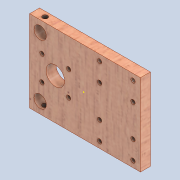
# Autodesk Inventor part: 0005-10-011
Saved by Autodesk Inventor 2020 (Build 240168000, 168)
## iProperties
Created: 2020-12-18
Part Number: 0005-10-011
Material: Wood (Maple)
Document SubType Name: Modeling
Designer: Iulian Bors
Density: 0.67 g/cm^3
Appearance: White Oak - Natural Medium Gloss
Mass: 29.1797 g
Surface Area: 153.939 cm^2
Volume: 43.5518 cm^3
Author: Iulian Bors
Subject: 011
Autodesk Inventor part; units mm, degrees
ref_plane "YZ Plane" through (0, 0, 0) normal (1, 0, 0) x (0, 1, 0)
ref_plane "XZ Plane" through (0, 0, 0) normal (0, 1, 0) x (-1, 0, 0)
ref_plane "XY Plane" through (0, 0, 0) normal (0, 0, 1) x (1, 0, 0)
sketch "Sketch1" plane through (0, 0, 0) normal (0, 0, 1) x (1, 0, 0)
  line L0 (-43.75, 33) -> (43.75, 33)
  line L1 (43.75, 33) -> (43.75, -33)
  line L2 (43.75, -33) -> (-43.75, -33)
  line L3 (-43.75, -33) -> (-43.75, 33)
  point P0 (0, 0)
  point P1 (0, 33)
  point P2 (-43.75, 0)
  dimension "d0" = 87.5
  dimension "d1" = 66
  constraints: 8 end point, 2 midpoint, 2 parallel, 1 horizontal, 1 horizontal alignment, 1 perpendicular, 1 vertical alignment
  measures "d0" distance of L0.start L0.end
  measures "d1" distance of L2.end L0.start
extrude "Extrusion1" add sketch "Sketch1" along normal blind 8
sketch "Sketch4" plane through (0, 0, 8) normal (0, 0, 1) x (1, 0, 0)
  line L0 (43.75, 33) -> (-43.75, 33) projected
  line L1 (-43.75, 33) -> (-43.75, -33) projected
  circle A0 centre (-35.25, 24) radius 5
  circle A1 centre (-35.25, -24) radius 5
  line L2 (-43.75, -33) -> (43.75, -33) projected
  point P0 (0, 0)
  dimension "d27" = 8.5
  dimension "d28" = 9
  dimension "d29" = 10
  dimension "d30" = 9
  constraints: 2 centre point, 1 equal radius, 1 vertical alignment
  measures "d27" distance from line of A0.centre L1
  measures "d28" distance from line of L0 A0.centre
  measures "d29" diameter of A0
  measures "d30" distance from line of L2 A1.centre
extrude "Extrusion4" cut sketch "Sketch4" against normal through all
sketch "Sketch5" plane through (0, 0, 8) normal (0, 0, 1) x (1, 0, 0)
  circle A0 centre (-23.0012, 0) radius 4
  circle A1 centre (-23.0012, 0) radius 7.5
  line L0 (-43.75, 33) -> (-43.75, -33) projected
  line L1 (43.75, 33) -> (-43.75, 33) projected
  circle A2 centre (-23.0012, 0) radius 7 projected
  point P0 (0, 0)
  point P1 (-43.75, 0)
  dimension "d24" = 15
  dimension "d33" = 20.7488
  constraints: 2 centre point, 2 horizontal alignment, 1 concentric, 1 midpoint
  measures "d24" diameter of A1
  measures "d33" distance from line of A0.centre L0
extrude "Extrusion5" cut sketch "Sketch5" against normal through all contours A0 | A1 | A2
sketch "Sketch6" plane through (0, 0, 8) normal (0, 0, 1) x (1, 0, 0)
  circle A0 centre (-33.7512, 10) radius 1.75
  circle A1 centre (-12.2512, 10) radius 1.75
  circle A2 centre (-12.2512, -10) radius 1.75
  circle A3 centre (-33.7512, -10) radius 1.75
  line L0 (-33.7512, 10) -> (-12.2512, 10)
  line L1 (-12.2512, 10) -> (-12.2512, -10)
  line L2 (-12.2512, -10) -> (-33.7512, -10)
  line L3 (-33.7512, -10) -> (-33.7512, 10)
  line L4 (-33.7512, 10) -> (-12.2512, -10) construction
  line L5 (-12.2512, 10) -> (-33.7512, -10) construction
  circle A4 centre (-23.0012, 0) radius 7.5 projected
  line L6 (-43.75, 33) -> (-43.75, -33) projected
  point P0 (0, 0)
  point P1 (-23.0012, 0)
  dimension "d35" = 3.5
  dimension "d36" = 21.5
  dimension "d37" = 20
  constraints: 12 end point, 4 centre point, 4 coincident, 3 equal radius, 3 midpoint, 3 parallel, 1 horizontal
  measures "d35" diameter of A1
  measures "d36" distance of L0.start L0.end
  measures "d37" distance of L0.end L1.end
extrude "Extrusion6" cut sketch "Sketch6" against normal through all contours L0 L3 A0 | A0 L3 L0 | L0 L1 A1 | A1 L1 L0 | L3 L2 A3 | A3 L2 L3 | L1 L2 A2 | A2 L2 L1
sketch "Sketch7" plane through (0, 0, 8) normal (0, 0, 1) x (1, 0, 0)
  point P0 (0, 0)
sketch "Sketch8" plane through (0, 0, 0) normal (0, 0, -1) x (-1, 0, 0)
  line L0 (-35.75, -33) -> (-43.75, -33)
  line L1 (-43.75, -33) -> (-43.75, 33)
  line L2 (-43.75, 33) -> (-35.75, 33)
  line L3 (-35.75, 33) -> (-35.75, -33)
  line L4 (-8.75, -33) -> (-16.75, -33)
  line L5 (-16.75, -33) -> (-16.75, 33)
  line L6 (-16.75, 33) -> (-8.75, 33)
  line L7 (-8.75, 33) -> (-8.75, -33)
  line L8 (-44.55, -20.5) -> (-44.55, -29.5) projected
  point P0 (0, 0)
  point P1 (-39.75, -28)
  point P2 (-39.75, -13)
  point P3 (-39.75, 13)
  point P4 (-39.75, 28)
  dimension "d38" = 4
  dimension "d39" = 5
  dimension "d40" = 15
  dimension "d41" = 5
  dimension "d42" = 15
  dimension "d56" = 26
  constraints: 16 end point, 4 horizontal, 4 vertical, 3 vertical alignment, 8 other
  measures "d38" distance from line of point (-39.75, -13) L1
  measures "d39" distance from line of point (-39.75, -28) L0
  measures "d40" distance of point (-39.75, -28) point (-39.75, -13)
  measures "d41" distance from line of point (-39.75, 28) L2
  measures "d42" distance of point (-39.75, 28) point (-39.75, 13)
  measures "d56" distance of point (-39.75, -13) point (-39.75, 13)
hole "Hole1" at (39.75, 28, 0) direction (0, 0, 1) diameter 3.5 end through all
move faces "Move1" translate (2, 0, 0) faces at (43.75, -11, 2.6667)
pattern_linear "Rectangular Pattern2" count 2 spacing 15 along (0, -1, 0) count 2 spacing 41 along (0, -1, 0) of "Hole1"
pattern_linear "Rectangular Pattern3" count 2 spacing 27 along (-1, 0, 0) of "Hole1", "Rectangular Pattern2"
sketch "Sketch10" plane through (-43.75, 33, 8) normal (0, 1, 0) x (1, 0, 0)
  line L0 (0, 8) -> (0, 0) projected
  point P0 (43.75, 8)
  point P1 (8.5, 4)
  point P2 (0, 4)
  dimension "d66" = 8.5
  constraints: 1 horizontal alignment, 1 midpoint
  measures "d66" distance from line of L0 point (8.5, 4)
hole "Hole2" at (-35.25, 33, 4) direction (0, -1, 0) diameter 4.134 depth 7.45 tip angle 118 thread size "M5x0.8" class "6H" standard "ISO Metric profile"
sketch "Sketch11" plane through (-43.75, -33, 0) normal (0, -1, 0) x (1, 0, 0)
  line L0 (0, 0) -> (0, 8) projected
  point P0 (43.75, 0)
  point P1 (8.5, 4)
  point P2 (0, 4)
  dimension "d74" = 8.5
  constraints: 1 horizontal alignment, 1 midpoint
  measures "d74" distance from line of L0 point (8.5, 4)
hole "Hole3" at (-35.25, -33, 4) direction (0, 1, 0) diameter 4.134 depth 7.45 tip angle 118 thread size "M5x0.8" class "6H" standard "ISO Metric profile"
equation "\"d30\" = d28"
equation "\"d41\" = d39"
equation "\"d42\" = d40"
body "Solid1"
